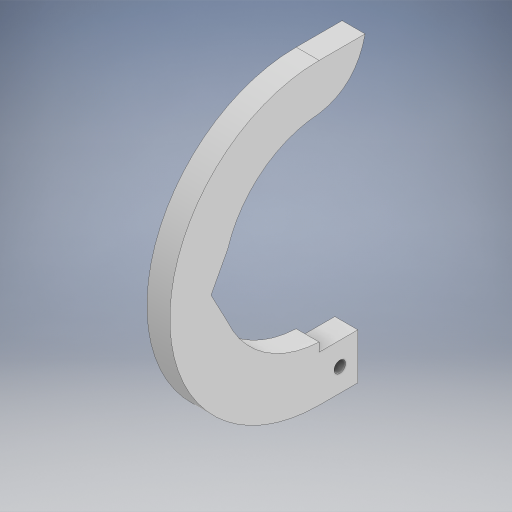
# Autodesk Inventor part: hook3
Saved by Autodesk Inventor 2024.2 (Build 282272000, 272)
## iProperties
Created: 2024-03-12
Part Number: hook3
Material: Generic
Document SubType Name: Modeling
Designer: rohan
Density: 1 g/cm^3
Appearance: Default
Author: rohan
Autodesk Inventor part; units mm, degrees
ref_plane "YZ Plane" through (0, 0, 0) normal (1, 0, 0) x (0, 1, 0)
ref_plane "XZ Plane" through (0, 0, 0) normal (0, 1, 0) x (-1, 0, 0)
ref_plane "XY Plane" through (0, 0, 0) normal (0, 0, 1) x (1, 0, 0)
sketch "Sketch1" plane through (0, 0, 0) normal (1, 0, 0) x (0, 1, 0)
  line L0 (-79.087, -26.0411) -> (-53.687, -26.0411)
  line L1 (-79.087, -47.4154) -> (-53.687, -47.4154)
  arc A0 (86.013, -26.0411) -> (-79.087, -26.0411) centre (3.463, -26.0411) ccw
  line L2 (86.013, -26.0411) -> (86.013, -51.4411)
  line L3 (60.613, -26.0411) -> (64.0729, -46.4736) construction
  line L4 (64.0729, -46.4736) -> (86.013, -51.4411) construction
  spline S0 degree 2 poles (60.613, -26.0411) (64.0729, -46.4736) (86.013, -51.4411) knots 1 1 1 2 2 2
  line L5 (-79.087, -26.0411) -> (-79.087, -47.4154)
  line L6 (-53.687, -26.0411) -> (-53.687, -47.4154)
  circle A1 centre (-66.387, -37.4662) radius 3.175
  line L7 (3.463, 33.7573) -> (8.9784, 30.8422)
  line L8 (3.463, 33.7573) -> (-2.0524, 30.8422)
  line L9 (-2.0524, 30.8422) -> (-14.0246, 24.5144)
  line L10 (8.9784, 30.8422) -> (20.9506, 24.5144)
  arc A2 (60.613, -26.0411) -> (20.9506, 24.5144) centre (4.4241, -29.2871) ccw
  arc A3 (-14.0246, 24.5144) -> (-48.843, -26.0411) centre (9.4259, -28.9041) ccw
  line L11 (-48.843, -26.0411) -> (-53.687, -26.0411)
  point P0 (0, 0)
  dimension "d0" = 114.3
  constraints: 20 end point, 6 point on circle, 4 centre point, 1 horizontal, 1 point on line, 3 other
  measures "d0" distance of L0.end L3.start
extrude "Extrusion2" add sketch "Sketch1" along normal blind 12.7
body "Solid2"
